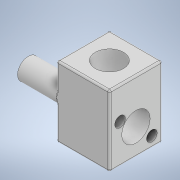
# Autodesk Inventor part: cantoneira
Saved by Autodesk Inventor 2022 (Build 260153000, 153)
## iProperties
Created: 2022-02-16
Part Number: cantoneira
Material: Genérico
Document SubType Name: Modeling
Designer: mathe
Density: 1 g/cm^3
Appearance: Padrão
Author: mathe
Autodesk Inventor part; units mm, degrees
ref_plane "YZ Plane" through (0, 0, 0) normal (1, 0, 0) x (0, 1, 0)
ref_plane "XZ Plane" through (0, 0, 0) normal (0, 1, 0) x (-1, 0, 0)
ref_plane "XY Plane" through (0, 0, 0) normal (0, 0, 1) x (1, 0, 0)
sketch "Esboço1" plane through (0, 0, 0) normal (0, 1, 0) x (-1, 0, 0)
  line L0 (0, 0) -> (15, 0)
  line L1 (15, 0) -> (15, -15)
  line L2 (15, -15) -> (0, -15)
  line L3 (0, -15) -> (0, 0)
  dimension "d0" = 15
  dimension "d1" = 15
  constraints: 8 end point, 2 parallel, 1 horizontal, 1 perpendicular
  measures "d0" distance of L1.end L2.end
  measures "d1" distance of L0.end L1.end
extrude "Extrusão1" add sketch "Esboço1" along normal blind 20
sketch "Esboço2" plane through (0, 0, 0) normal (1, 0, 0) x (0, 0, -1)
  point P0 (0, 0)
  point P1 (7.5, 7.5)
hole "Furo1" at (0, 7.5, -7.5) direction (-1, 0, 0) diameter 8 depth 12
sketch "Esboço4" plane through (0, 20, 0) normal (0, 1, 0) x (1, 0, 0)
  point P0 (0, 0)
  point P1 (-7.5, 7.5)
hole "Furo2" at (-7.5, 20, -7.5) direction (0, -1, 0) diameter 8 depth 7.5
sketch "Esboço5" plane through (0, 0, 0) normal (1, 0, 0) x (0, 0, -1)
  circle A0 centre (3, 11) radius 1.5
  circle A1 centre (12, 3) radius 1.5
  point P0 (0, 0)
  dimension "d19" = 3
  dimension "d20" = 3
  constraints: 2 centre point, 2 coincident
  measures "d19" diameter of A0
  measures "d20" diameter of A1
extrude "Extrusão2" cut sketch "Esboço5" against normal through all
sketch "Esboço6" plane through (-15, 0, -15) normal (-1, 0, 0) x (0, 0, 1)
  circle A0 centre (3, 3) radius 1.5 projected
  circle A1 centre (3, 3) radius 3
  circle A2 centre (12, 11) radius 1.5 projected
  circle A3 centre (12, 11) radius 3
  point P0 (15, 0)
  dimension "d23" = 6
  dimension "d24" = 6
  constraints: 2 centre point, 2 coincident
  measures "d23" diameter of A1
  measures "d24" diameter of A3
extrude "Extrusão3" add sketch "Esboço6" along normal blind 11
fillet "Arredondamento2" radius 0.5 15 edges at (-15, 11.5, -15) (-15, 1.5, -15) (-15, 0, -13.5) (-15, 0, -6) (-7.5, 0, -15) (-7.5, 0, 0) (-15, 5.5, 0) (-15, 15.5, 0) (-7.5, 20, 0) (-15, 20, -7.5) (-7.5, 20, -15) (0, 20, -7.5) (0, 10, -15) (0, 0, -7.5) (0, 10, 0)
